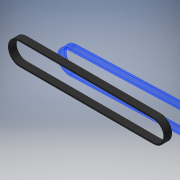
# Autodesk Inventor part: 30-30-750-HTD5M
Saved by Autodesk Inventor 2019.4 (Build 234330000, 330)
## iProperties
Created: 2020-01-05
Part Number: 30-30-750-HTD5M
Material: Rubber
Document SubType Name: Modeling
Designer: Mark
Mass: 37.5709 g
Surface Area: 278.303 cm^2
Volume: 40.3988 cm^3
Density: 0.93 g/cm^3
Appearance: Rubber - Black
Author: Mark
Autodesk Inventor part; units mm, degrees
ref_plane "YZ Plane" through (0, 0, 0) normal (1, 0, 0) x (0, 1, 0)
ref_plane "XZ Plane" through (0, 0, 0) normal (0, 1, 0) x (-1, 0, 0)
ref_plane "XY Plane" through (0, 0, 0) normal (0, 0, 1) x (1, 0, 0)
sketch "Sketch1" plane through (0, 0, 0) normal (0, 0, 1) x (1, 0, 0)
  arc A0 (0, 23.875) -> (0, -23.875) centre (0, 0) ccw
  arc A1 (290, -23.875) -> (290, 23.875) centre (290, 0) ccw
  line L0 (0, 23.875) -> (290, 23.875)
  line L1 (290, -23.875) -> (0, -23.875)
  line L2 (290, 21.775) -> (0, 21.775)
  arc A2 (0, 21.775) -> (0, -21.775) centre (0, 0) ccw
  line L3 (0, -21.775) -> (290, -21.775)
  arc A3 (290, -21.775) -> (290, 21.775) centre (290, 0) ccw
  line L4 (290, 25.375) -> (0, 25.375)
  arc A4 (0, 25.375) -> (0, -25.375) centre (0, 0) ccw
  line L5 (0, -25.375) -> (290, -25.375)
  arc A5 (290, -25.375) -> (290, 25.375) centre (290, 0) ccw
  dimension "d0" = 47.75
  dimension "d1" = 47.75
  dimension "d2" = 290
  dimension "d3" = 2.1
  dimension "d4" = 1.5
  constraints: 12 end point, 12 point on circle, 6 centre point, 4 tangent, 1 coincident, 6 other
  measures "d0" diameter of A0
  measures "d1" diameter of A1
  measures "d2" distance of A0.centre A1.centre
  measures "d3" distance between parallel lines of L0 L2
  measures "d4" distance between parallel lines of L0 L4
extrude "Extrusion1" add sketch "Sketch1" along normal blind 15 contours L0 A1 L1 A0 | A5 L5 A4 L4
body "Solid1"
